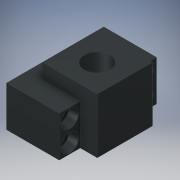
# Autodesk Inventor part: Festlager
Saved by Autodesk Inventor 2019 (Build 230136000, 136)
## iProperties
Created: 2021-04-25
Part Number: Festlager
Material: Eisen, Grau
Document SubType Name: Modeling
Designer: Michael Sumper
Density: 7.15 g/cm^3
Appearance: Eisen - Grau
Author: Michael Sumper
Autodesk Inventor part; units mm, degrees
ref_plane "YZ Plane" through (0, 0, 0) normal (1, 0, 0) x (0, 1, 0)
ref_plane "XZ Plane" through (0, 0, 0) normal (0, 1, 0) x (-1, 0, 0)
ref_plane "XY Plane" through (0, 0, 0) normal (0, 0, 1) x (1, 0, 0)
sketch "Skizze1" plane through (0, 0, 0) normal (1, 0, 0) x (0, 1, 0)
  line L0 (-12.5, 30) -> (12.5, 30)
  line L1 (12.5, 30) -> (12.5, -30)
  line L2 (12.5, -30) -> (-12.5, -30)
  line L3 (-12.5, -30) -> (-12.5, 30)
  line L4 (-12.5, 30) -> (12.5, -30) construction
  line L5 (12.5, 30) -> (-12.5, -30) construction
  point P0 (0, 0)
  dimension "d0" = 25
  dimension "d1" = 60
  constraints: 12 end point, 2 midpoint, 2 parallel, 1 horizontal, 1 perpendicular
  measures "d0" distance of L1.end L2.end
  measures "d1" distance of L0.end L1.end
extrude "Extrusion1" add sketch "Skizze1" along normal blind 32.5
sketch "Skizze2" plane through (32.5, 0, 0) normal (1, 0, 0) x (0, 0, -1)
  line L0 (-30, -12.5) -> (30, -12.5) construction
  line L1 (0, -12.5) -> (17, -12.5) construction
  line L2 (17, -12.5) -> (-17, -12.5)
  line L3 (-17, -12.5) -> (-17, 21.5)
  line L4 (-17, 21.5) -> (17, 21.5)
  line L5 (17, 21.5) -> (17, -12.5)
  point P0 (0, 0)
  dimension "d4" = 17
  dimension "d5" = 34
  dimension "d6" = 34
  constraints: 10 end point, 2 parallel, 1 horizontal, 1 midpoint, 1 perpendicular, 1 point on line
  measures "d4" distance of L1.start L1.end
  measures "d5" distance of L3.end L4.end
  measures "d6" distance of L2.end L3.end
extrude "Extrusion2" add sketch "Skizze2" along normal blind 10.5
extrude "Extrusion3" add sketch "Skizze2" against normal blind 23.5
sketch "Skizze3" plane through (43, 21.5, 17) normal (0, 1, 0) x (1, 0, 0)
  line L0 (-34, 0) -> (-34, 34) construction
  line L1 (-10.5, 34) -> (0, 34) construction
  line L2 (-34, 0) -> (0, 34) construction
  line L3 (0, 34) -> (0, 0) construction
  line L4 (-34, 34) -> (0, 0) construction
  point P0 (-43, 17)
  constraints: 4 end point
sketch "Skizze4" plane through (43, 21.5, 17) normal (0, 1, 0) x (1, 0, 0)
  point P0 (-43, 17)
  point P1 (-17, 17)
hole "Bohrung1" at (26, 21.5, 0) direction (0, -1, 0) diameter 16 end through all
sketch "Skizze5" plane through (32.5, 0, 0) normal (1, 0, 0) x (0, 0, -1)
  line L0 (-17, 21.5) -> (-17, -12.5) construction
  line L1 (-17, 12.5) -> (-30, 12.5) construction
  line L2 (-30, 12.5) -> (-30, -12.5) construction
  line L3 (-30, -12.5) -> (-17, -12.5) construction
  line L4 (-30, 12.5) -> (30, 12.5) construction
  line L5 (-23.5, 12.5) -> (-23.5, -12.5) construction
  line L6 (30, -12.5) -> (-30, -12.5) construction
  line L7 (-23.5, 12.5) -> (-23.5, 6.5) construction
  line L8 (-23.5, 6.5) -> (-23.5, -6.5) construction
  line L9 (-23.5, 6.5) -> (22.5, 6.5) construction
  line L10 (22.5, 6.5) -> (22.5, -6.5) construction
  point P0 (0, 0)
  dimension "d18" = 6
  dimension "d19" = 13
  dimension "d20" = 46
  dimension "d21" = 13
  constraints: 10 end point, 4 point on line, 2 perpendicular, 1 horizontal
  measures "d18" distance of L5.start L7.end
  measures "d19" distance of L7.end L8.end
  measures "d20" distance of L7.end L9.end
  measures "d21" distance of L9.end L10.end
hole "Bohrung2" at (32.5, 6.5, 23.5) at (32.5, -6.5, 23.5) at (32.5, 6.5, -22.5) at (32.5, -6.5, -22.5) direction (-1, 0, 0) diameter 6.6 end through all counterbore diameter 11 counterbore depth 6 clearance for "Innensechskantkopfschraube" size "M6" standard "ANSI Metrisches M Profil"
